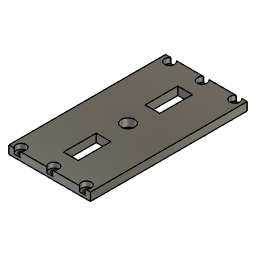
Unified Pivot Base v8 (Autodesk Fusion 360 design; units mm, degrees)
Autodesk Fusion 360 part; units mm, degrees
sketch "Schizzo5" plane through (0, 0, 0) normal (0, 0, 1) x (1, 0, 0)
  line L0 (84.3315, 82.4519) -> (84.3315, -13.5481)
  circle A0 centre (89.3315, -11.0481) radius 1.5
  circle A1 centre (129.3315, 79.9519) radius 3
  line L1 (84.3315, 34.4519) -> (134.3315, 34.4519) construction
  circle A2 centre (109.3315, 79.9519) radius 1.5
  circle A3 centre (89.3315, 79.9519) radius 3
  circle A4 centre (89.3315, 79.9519) radius 1.5
  line L2 (134.3315, 82.4519) -> (84.3315, 82.4519)
  circle A5 centre (129.3315, 79.9519) radius 1.5
  circle A6 centre (109.3315, 79.9519) radius 3
  circle A7 centre (109.3315, 34.4519) radius 4.1
  circle A8 centre (109.3315, -11.0481) radius 1.5
  line L3 (134.3315, -13.5481) -> (134.3315, 82.4519)
  line L4 (89.3315, 82.4519) -> (89.3315, -13.5481) construction
  circle A9 centre (89.3315, -11.0481) radius 3
  circle A10 centre (109.3315, -11.0481) radius 3
  circle A11 centre (129.3315, -11.0481) radius 1.5
  line L5 (84.3315, -13.5481) -> (134.3315, -13.5481)
  circle A12 centre (129.3315, -11.0481) radius 3
  line L6 (84.3315, -11.0481) -> (134.3315, -11.0481) construction
  line L7 (109.3315, 82.4519) -> (109.3315, -13.5481) construction
  line L8 (109.3315, 34.4519) -> (109.3315, 59.4519) construction
  line L9 (113.8315, -0.5481) -> (104.8315, -0.5481)
  line L10 (104.8315, -0.5481) -> (104.8315, 19.4519)
  line L11 (104.8315, 19.4519) -> (113.8315, 19.4519)
  line L12 (113.8315, 19.4519) -> (113.8315, -0.5481)
  line L13 (113.8315, -0.5481) -> (104.8315, 19.4519) construction
  line L14 (104.8315, -0.5481) -> (113.8315, 19.4519) construction
  line L15 (113.8315, 49.4519) -> (113.8315, 69.4519)
  line L16 (104.8315, 49.4519) -> (113.8315, 49.4519)
  line L17 (104.8315, 69.4519) -> (104.8315, 49.4519)
  line L18 (113.8315, 69.4519) -> (104.8315, 69.4519)
  line L19 (104.8315, 69.4519) -> (113.8315, 49.4519) construction
  line L20 (113.8315, 69.4519) -> (104.8315, 49.4519) construction
  point P0 (127.8474, 12.2366)
  point P1 (109.3315, 9.4519)
  point P2 (109.3315, 59.4519)
  dimension "d221" = 50
  dimension "d222" = 96
  dimension "d223" = 2.5
  dimension "d224" = 20
  dimension "d225" = 3
  dimension "d226" = 6
  dimension "d227" = 3
  dimension "d228" = 6
  dimension "d229" = 8.2
  dimension "d354" = 9
  dimension "d355" = 20
  dimension "d356" = 50
  constraint horizontal L5
  constraint vertical L3
  constraint horizontal L2
  constraint vertical L0
  constraint midpoint L7.start L2
  constraint midpoint L7.end L5
  constraint coincident L6.end L3
  constraint perpendicular L3 L6
  constraint midpoint L1.start L0
  constraint midpoint L1.end L3
  constraint coincident L4.start L2
  constraint coincident L4.end L5
  constraint perpendicular L4 L5
  constraint coincident A0.centre L6
  constraint coincident A0.centre L4
  constraint concentric A0 A9
  constraint symmetric A0 A11 L7
  constraint symmetric A9 A12 L7
  constraint symmetric A0 L1 A4
  constraint symmetric L1 A3 A9
  constraint symmetric L1 A5 A11
  constraint symmetric A1 L1 A12
  constraint coincident A8.centre L7
  constraint coincident A8.centre L6
  constraint concentric A8 A10
  constraint symmetric L1 A2 A8
  constraint symmetric L1 A6 A10
  constraint midpoint A7.centre L1
  constraint coincident P2 L7
  constraint coincident L6.start L0
  constraint horizontal L9
  constraint perpendicular L9 L10
  constraint parallel L9 L11
  constraint parallel L10 L12
  constraint coincident L13 P1
  constraint coincident L14 P1
  constraint coincident L7 P1
  constraint symmetric L1 L9.start L15.end
  constraint symmetric L1 L9.end L17.start
  constraint symmetric L1 L10.end L16.start
  constraint symmetric L1 L11.end L15.start
  constraint symmetric L1 P1 P2
  measures "d221" distance of L0.end L3.start
  measures "d222" distance of L0.end L0.start
  measures "d223" distance of L5 L6
  measures "d224" distance of L4 L7
  measures "d225" diameter of A0
  measures "d226" diameter of A9
  measures "d227" diameter of A8
  measures "d228" diameter of A10
  measures "d229" diameter of A7
  measures "d354" distance of L10.end L11.end
  measures "d355" distance of L9.end L10.end
  measures "d356" distance of P1 P2
extrude "Estrusione24" add sketch "Schizzo5" along normal blind 5 contours L0 A1 A3 L2 A6 L3 A9 A10 L5 A12 | A3 L2 | A9 L5 | L2 A6 | A10 L5 | A1 L2 | L5 A12 picked at (89.3689, 82.1172) picked at (89.3689, -13.2134) picked at (109.3689, 82.1172) picked at (109.3689, -13.2134) picked at (129.3689, 82.1172) picked at (129.3689, -13.2134)
extrude "Estrusione25" cut sketch "Schizzo5" against normal blind 3.2 from surface at 5 contours A3 L2 | A9 L5 | L2 A6 | A10 L5 | A1 L2 | L5 A12 picked at (89.3689, 82.1172) picked at (89.3689, -13.2134) picked at (109.3689, 82.1172) picked at (109.3689, -13.2134) picked at (129.3689, 82.1172) picked at (129.3689, -13.2134)
equation "d225 = d227"
equation "d226 = d228"
named bodies: "Base"
